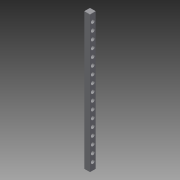
# Autodesk Inventor part: pole
Saved by Autodesk Inventor 2015 (Build 190159000, 159)
## iProperties
Created: 2015-01-15
Part Number: pole
Material: Generic
Document SubType Name: Modeling
Designer: Tucker
Density: 1 g/cm^3
Appearance: Default
Author: Tucker
Autodesk Inventor part; units mm, degrees
ref_plane "YZ Plane" through (0, 0, 0) normal (1, 0, 0) x (0, 1, 0)
ref_plane "XZ Plane" through (0, 0, 0) normal (0, 1, 0) x (-1, 0, 0)
ref_plane "XY Plane" through (0, 0, 0) normal (0, 0, 1) x (1, 0, 0)
sketch "Sketch1" plane through (0, 0, 0) normal (1, 0, 0) x (0, 1, 0)
  line L0 (0, 0) -> (1828.8, 0)
  line L1 (1828.8, 0) -> (1828.8, -76.2)
  line L2 (1828.8, -76.2) -> (0, -76.2)
  line L3 (0, -76.2) -> (0, 0)
  dimension "d0" = 1828.8
  dimension "d1" = 76.2
  constraints: 8 end point, 2 parallel, 1 horizontal, 1 perpendicular
  measures "d0" distance of L1.end L2.end
  measures "d1" distance of L0.end L1.end
extrude "Extrusion1" add sketch "Sketch1" along normal blind 76.2
sketch "Sketch2" plane through (76.2, 0, 0) normal (1, 0, 0) x (0, 0, -1)
  circle A0 centre (38.1, 101.6) radius 25.4
  circle A1 centre (38.1, 203.2) radius 25.4
  circle A2 centre (38.1, 304.8) radius 25.4
  circle A3 centre (38.1, 406.4) radius 25.4
  circle A4 centre (38.1, 508) radius 25.4
  circle A5 centre (38.1, 609.6) radius 25.4
  circle A6 centre (38.1, 711.2) radius 25.4
  circle A7 centre (38.1, 812.8) radius 25.4
  circle A8 centre (38.1, 914.4) radius 25.4
  circle A9 centre (38.1, 1016) radius 25.4
  circle A10 centre (38.1, 1117.6) radius 25.4
  circle A11 centre (38.1, 1219.2) radius 25.4
  circle A12 centre (38.1, 1320.8) radius 25.4
  circle A13 centre (38.1, 1422.4) radius 25.4
  circle A14 centre (38.1, 1524) radius 25.4
  circle A15 centre (38.1, 1625.6) radius 25.4
  circle A16 centre (38.1, 1727.2) radius 25.4
  point P0 (0, 0)
  dimension "d4" = 50.8
  dimension "d5" = 50.8
  dimension "d6" = 50.8
  dimension "d7" = 50.8
  dimension "d8" = 50.8
  dimension "d9" = 50.8
  dimension "d10" = 50.8
  dimension "d11" = 50.8
  dimension "d12" = 50.8
  dimension "d13" = 50.8
  dimension "d14" = 50.8
  dimension "d15" = 50.8
  dimension "d16" = 50.8
  dimension "d17" = 50.8
  dimension "d18" = 50.8
  dimension "d19" = 50.8
  dimension "d20" = 50.8
  constraints: 17 centre point
  measures "d4" diameter of A0
  measures "d5" diameter of A1
  measures "d6" diameter of A2
  measures "d7" diameter of A3
  measures "d8" diameter of A4
  measures "d9" diameter of A5
  measures "d10" diameter of A6
  measures "d11" diameter of A7
  measures "d12" diameter of A8
  measures "d13" diameter of A9
  measures "d14" diameter of A10
  measures "d15" diameter of A11
  measures "d16" diameter of A12
  measures "d17" diameter of A13
  measures "d18" diameter of A14
  measures "d19" diameter of A15
  measures "d20" diameter of A16
extrude "Extrusion2" cut sketch "Sketch2" against normal blind 127
body "Solid1"
